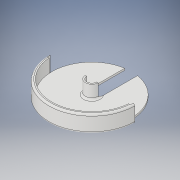
# Autodesk Inventor part: casept1
Saved by Autodesk Inventor 2018 (Build 220112000, 112)
## iProperties
Created: 2018-03-21
Part Number: casept1
Material: PC/ABS Plastic
Document SubType Name: Modeling
Designer: FablabGuest
Density: 0.357273 g/cm^3
Appearance: Smooth - White
Author: FablabGuest
Autodesk Inventor part; units mm, degrees
ref_plane "YZ Plane" through (0, 0, 0) normal (1, 0, 0) x (0, 1, 0)
ref_plane "XZ Plane" through (0, 0, 0) normal (0, 1, 0) x (-1, 0, 0)
ref_plane "XY Plane" through (0, 0, 0) normal (0, 0, 1) x (1, 0, 0)
sketch "Sketch1" plane through (0, 0, 0) normal (0, 1, 0) x (-1, 0, 0)
  circle A0 centre (0, 0) radius 70
  dimension "d0" = 140
  constraints: 1 centre point, 1 coincident
  measures "d0" diameter of A0
extrude "Extrusion1" add sketch "Sketch1" along normal blind 28
sketch "Sketch2" plane through (0, 28, 0) normal (0, 1, 0) x (1, 0, 0)
  circle A0 centre (0, 0) radius 8.25
  dimension "d3" = 16.5
  constraints: 1 centre point, 1 coincident
  measures "d3" diameter of A0
extrude "Extrusion2" cut sketch "Sketch2" against normal blind 280
sketch "Sketch3" plane through (0, 28, 0) normal (0, 1, 0) x (1, 0, 0)
  circle A0 centre (0, 0) radius 8.25 projected
  circle A1 centre (0, 0) radius 65
  circle A2 centre (0, 0) radius 10.5
  dimension "d6" = 130
  dimension "d7" = 21
  constraints: 2 centre point, 2 coincident
  measures "d6" diameter of A1
  measures "d7" diameter of A2
extrude "Extrusion3" cut sketch "Sketch3" against normal blind 22 contours A1
sketch "Sketch4" plane through (0, 6, 0) normal (0, 1, 0) x (1, 0, 0)
  line L0 (-77.4845, 0) -> (88.5537, 0)
  line L1 (88.5537, 0) -> (88.5537, 100.8261)
  line L2 (88.5537, 100.8261) -> (-77.4845, 100.8261)
  line L3 (-77.4845, 100.8261) -> (-77.4845, 0)
  point P0 (0, 0)
  constraints: 8 end point, 2 parallel, 1 horizontal, 1 perpendicular
extrude "Extrusion4" cut sketch "Sketch4" along normal blind 220
sketch "Sketch5" plane through (0, 0, 0) normal (0, -1, 0) x (1, 0, 0)
  circle A0 centre (0, 0) radius 8.25 projected
  circle A1 centre (0, 0) radius 70
  constraints: 1 centre point, 1 coincident
extrude "Extrusion5" cut sketch "Sketch5" against normal blind 3
sketch "Sketch6" plane through (0, 6, 0) normal (0, 1, 0) x (1, 0, 0)
  arc A0 (-65, 0) -> (65, 0) centre (0, 0) ccw projected
  line L0 (65, 0) -> (70, 0) projected
  arc A1 (70, 0) -> (-70, 0) centre (0, 0) ccw projected
  line L1 (-70, 0) -> (-65, 0) projected
  arc A2 (-10.5, 0) -> (10.5, 0) centre (0, 0) ccw projected
  line L2 (-10.5, 0) -> (-8.25, 0) projected
  arc A3 (8.25, 0) -> (-8.25, 0) centre (0, 0) ccw projected
  line L3 (8.25, 0) -> (10.5, 0) projected
  circle A4 centre (0, 0) radius 8.25 projected
  arc A5 (65, 0) -> (-65, 0) centre (0, 0) ccw
  line L4 (-65, 0) -> (-70, 0)
  line L5 (65, 0) -> (70, 0)
  arc A6 (70, 0) -> (-70, 0) centre (0, 0) ccw projected
  arc A7 (70, 0) -> (70, 0) centre (0, 0) ccw
  constraints: 4 end point, 3 point on circle, 2 coincident, 2 horizontal, 1 centre point, 1 horizontal alignment, 3 other
extrude "Extrusion6" cut sketch "Sketch6" against normal blind 3 contours L1 A1 L0 A5
sketch "Sketch7" plane through (0, 3, 0) normal (0, -1, 0) x (1, 0, 0)
  point P0 (0, 0)
sketch "Sketch8" plane through (0, 3, 0) normal (0, -1, 0) x (1, 0, 0)
  arc A0 (65, 0) -> (-65, 0) centre (0, 0) ccw projected
  arc A1 (70, 0) -> (-70, 0) centre (0, 0) ccw projected
  arc A2 (70, 0) -> (-70, 0) centre (0, 0) ccw
  arc A3 (65, 0) -> (-65, 0) centre (0, 0) ccw
  line L0 (65, 0) -> (70, 0) projected
  line L1 (70, 0) -> (65, 0)
  line L2 (-65, 0) -> (-70, 0) projected
  line L3 (-65, 0) -> (-70, 0)
  constraints: 4 end point, 4 point on circle, 2 centre point, 2 coincident, 2 horizontal
extrude "Extrusion7" add sketch "Sketch8" along normal blind 3
sketch "Sketch9" plane through (0, 28, 0) normal (0, 1, 0) x (1, 0, 0)
  line L0 (10.5, 0) -> (-10.497, 0)
  line L1 (-10.497, 0) -> (-10.497, 68.6752)
  line L2 (-10.497, 68.6752) -> (10.5, 68.6752)
  line L3 (10.5, 68.6752) -> (10.5, 0)
  point P0 (0, 0)
  constraints: 8 end point, 2 parallel, 1 horizontal, 1 perpendicular
extrude "Extrusion8" cut sketch "Sketch9" against normal blind 30
sketch "Sketch10" plane through (0, 3, 0) normal (0, -1, 0) x (1, 0, 0)
  arc A0 (8.25, 0) -> (-8.25, 0) centre (0, 0) ccw projected
  arc A1 (8.25, 0) -> (-8.25, 0) centre (0, 0) ccw
  line L0 (8.25, 0) -> (8.25, 64.4743)
  arc A2 (65, 0) -> (-65, 0) centre (0, 0) ccw projected
  line L1 (-8.25, 0) -> (-8.25, 64.4743)
  arc A3 (8.25, 64.4743) -> (-8.25, 64.4743) centre (0, 0) ccw
  point P0 (8.2498, 0.0514)
  constraints: 5 point on circle, 4 end point, 2 centre point, 2 coincident, 2 vertical
extrude "Extrusion9" add sketch "Sketch10" along normal blind 3
sketch "Sketch11" plane through (0, 28, 0) normal (0, 1, 0) x (1, 0, 0)
  line L0 (70, 0) -> (65, 0) projected
  arc A0 (-65, 0) -> (-64.8074, -5) centre (0, 0) ccw
  line L1 (-67.6849, 0) -> (-65, 0)
  line L2 (-64.8074, -5) -> (-67.5, -5)
  arc A1 (-67.6849, 0) -> (-67.5, -5) centre (0, 0) ccw
  constraints: 4 end point, 4 point on circle, 2 centre point, 2 coincident, 1 parallel
extrude "Extrusion10" cut sketch "Sketch11" against normal blind 100
mirror "Mirror1" about plane through (0, 0, 0) normal (1, 0, 0) of "Extrusion10"
fillet "Fillet2" radius 3 1 edges at (0, 28, 70)
fillet "Fillet3" radius 3 1 edges at (0, 6, 10.5)
fillet "Fillet4" radius 3 1 edges at (0, 0, 70)
sketch "Sketch12" plane through (0, 6, 0) normal (0, 1, 0) x (1, 0, 0)
  line L0 (10.5, 64.1463) -> (10.5, 0) projected
  line L1 (10.5, 0) -> (13.5, 0)
  line L2 (13.5, 0) -> (13.5, 8.45)
  line L3 (13.5, 8.45) -> (10.5, 8.45)
  line L4 (10.5, 8.45) -> (10.5, 0)
  point P0 (0, 0)
  dimension "d31" = 8.45
  constraints: 8 end point, 2 parallel, 1 horizontal, 1 perpendicular
  measures "d31" distance of L2.end L1.end
extrude "Extrusion11" [suppressed]
sketch "Sketch13" plane through (10.5, 9, 0) normal (0, 0, 1) x (1, 0, 0)
  point P0 (-10.5, -9)
sketch "Sketch14" plane through (10.5, 9, 0) normal (0, 0, 1) x (1, 0, 0)
  line L0 (3, -3) -> (3, 0) projected
  line L1 (3, 0) -> (3, -3)
  line L2 (0, 0) -> (3, 0) projected
  line L3 (3, 0) -> (0, 0)
  arc A0 (0, 0) -> (3, -3) centre (3, 0) ccw
  point P0 (-10.5, -9)
  constraints: 4 end point, 2 point on circle, 1 centre point, 1 coincident, 1 collinear, 1 vertical
extrude "Extrusion12" [suppressed]
ref_plane "Work Plane2" through (-10.5, 9, 0) normal (1, 0, 0) x (0, 1, 0)
sketch "Sketch15" plane through (-10.5, 9, 0) normal (1, 0, 0) x (0, 1, 0)
  line L0 (64.1463, 3) -> (64.1463, 0)
  line L1 (0, 0) -> (-3, 0)
  spline S0 degree 3 poles (0, 0) (-0.6805, -1.2731) (-1.4339, -2.6712) (-2.5948, -5.5551) (-3, -7.0418) (-3, -8.4853) knots 0 0 0 0 0.433052 0.433052 0.866104 0.866104 0.866104 0.866104
  line L2 (64.1463, 3) -> (64.1463, 0)
  line L3 (-3, -8.4853) -> (-3, 0)
  line L4 (-3, 0) -> (0, 0) projected
  line L5 (0, 10.5) -> (0, 0) projected
  line L6 (0, 0) -> (-3, 0) projected
  line L7 (-3, 0) -> (-3, 13.5) projected
  line L8 (-3, 0) -> (0, 0) projected
  line L9 (19, 0) -> (0, 0) projected
  line L10 (-3, 0) -> (-6, 0) projected
  line L11 (0, 0) -> (-3, 0)
  line L12 (-3, 0) -> (-3, -8.4853)
  line L13 (-3, 0) -> (-3, -64.1468) projected
  point P0 (-9, 0)
  point P1 (0, -3)
  constraints: 12 end point, 1 collinear, 1 horizontal, 6 other
extrude "Extrusion13" add sketch "Sketch15" against normal blind 3
sketch "Sketch16" plane through (-13.5, 9, 0) normal (0, 0, 1) x (1, 0, 0)
  line L0 (3, 0) -> (0, 0)
  line L1 (0, 0) -> (0, -3)
  line L2 (3, -3) -> (3, 0)
  arc A0 (0, -3) -> (3, 0) centre (0, 0) ccw
  line L3 (3, 0) -> (0, 0) projected
  line L4 (0, -3) -> (0, 0) projected
  line L5 (0, 0) -> (0, -3)
  line L6 (0, 0) -> (3, 0)
  arc A1 (0, -3) -> (3, 0) centre (0, 0) ccw
  line L7 (13.5, -14.6065) -> (13.5, 24.6065) projected
  point P0 (13.5, -9)
  point P1 (-10.5, -9)
  constraints: 10 end point, 4 point on circle, 2 centre point, 2 collinear, 1 coincident, 1 vertical
revolve "Revolution1" cut sketch "Sketch16" angle 360 about axis through (0, -10, 0) along (0, 1, 0)
ref_plane "Work Plane3" through (-13.5, 7.5, 0) normal (0, 0, -1) x (-1, 0, 0)
sketch "Sketch17" plane through (-13.5, 7.5, 0) normal (0, 0, -1) x (-1, 0, 0)
  line L0 (0, 1.5) -> (-3, 1.5)
  arc A0 (-3, 1.5) -> (0, -1.5) centre (0, 1.5) ccw
  line L1 (0, 1.5) -> (-3, 1.5)
  arc A1 (-3, 1.5) -> (0, -1.5) centre (0, 1.5) ccw
  line L2 (0, -1.5) -> (2.6945, -1.5)
  line L3 (2.6945, -1.5) -> (2.6945, 1.5)
  line L4 (2.6945, 1.5) -> (0, 1.5)
  line L5 (2.6945, 1.5) -> (-3, 1.5)
  line L6 (2.6945, 1.5) -> (2.6945, -1.5)
  line L7 (-3.003, -1.5) -> (51.5, -1.5) projected
  line L8 (2.6945, -1.5) -> (0, -1.5)
  arc A2 (-3, 1.5) -> (0, -1.5) centre (0, 1.5) ccw
  line L9 (-13.5, -14.9009) -> (-13.5, 26.4056) projected
  point P0 (-13.5, -7.5)
  point P1 (13.5, -9)
  point P2 (-10.5, -9)
  point P3 (51.3074, -1.5)
  constraints: 16 end point, 7 point on circle, 3 centre point, 2 coincident, 2 perpendicular, 1 collinear, 1 horizontal, 1 vertical
revolve "Revolution2" cut sketch "Sketch17" angle 360 about axis through (0, -10, 0) along (0, 1, 0)
mirror "Mirror2" about plane through (0, 0, 0) normal (1, 0, 0) of "Extrusion13", "Revolution1", "Revolution2"
ref_plane "Work Plane1" through (0, 0, 0) normal (1, 0, 0) x (0, 1, 0)
body "Solid1"
